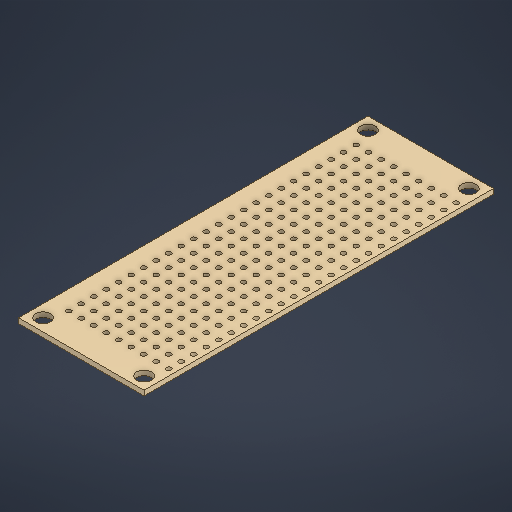
# Autodesk Inventor part: perfboard-71x51x1
Saved by Autodesk Inventor 2025.2 (Build 292293000, 293)
## iProperties
Created: 2025-11-15
Part Number: perfboard-71x51x1
Material: Fiberglass Batt
Document SubType Name: Modeling
Designer: sam
Density: 0.032 g/cm^3
Appearance: Golden Sand
Author: sam
Autodesk Inventor part; units mm, degrees
ref_plane "YZ Plane" through (0, 0, 0) normal (1, 0, 0) x (0, 1, 0)
ref_plane "XZ Plane" through (0, 0, 0) normal (0, 1, 0) x (-1, 0, 0)
ref_plane "XY Plane" through (0, 0, 0) normal (0, 0, 1) x (1, 0, 0)
sketch "Sketch1" plane through (0, 0, 0) normal (0, 1, 0) x (-1, 0, 0)
  line L0 (-12.75, -35.5) -> (12.75, -35.5)
  line L1 (12.75, -35.5) -> (12.75, 35.5)
  line L2 (12.75, 35.5) -> (-12.75, 35.5)
  line L3 (-12.75, 35.5) -> (-12.75, -35.5)
  line L4 (-12.75, -35.5) -> (12.75, 35.5) construction
  line L5 (12.75, -35.5) -> (-12.75, 35.5) construction
  circle A0 centre (8.84, -29.21) radius 0.5
  circle A1 centre (6.3, -29.21) radius 0.5
  circle A2 centre (3.76, -29.21) radius 0.5
  circle A3 centre (1.22, -29.21) radius 0.5
  circle A4 centre (-1.32, -29.21) radius 0.5
  circle A5 centre (-3.86, -29.21) radius 0.5
  circle A6 centre (-6.4, -29.21) radius 0.5
  circle A7 centre (-8.94, -29.21) radius 0.5
  circle A8 centre (-11.48, -29.21) radius 0.5
  circle A9 centre (8.84, -26.67) radius 0.5
  circle A10 centre (6.3, -26.67) radius 0.5
  circle A11 centre (3.76, -26.67) radius 0.5
  circle A12 centre (1.22, -26.67) radius 0.5
  circle A13 centre (-1.32, -26.67) radius 0.5
  circle A14 centre (-3.86, -26.67) radius 0.5
  circle A15 centre (-6.4, -26.67) radius 0.5
  circle A16 centre (-8.94, -26.67) radius 0.5
  circle A17 centre (-11.48, -26.67) radius 0.5
  circle A18 centre (8.84, -24.13) radius 0.5
  circle A19 centre (6.3, -24.13) radius 0.5
  circle A20 centre (3.76, -24.13) radius 0.5
  circle A21 centre (1.22, -24.13) radius 0.5
  circle A22 centre (-1.32, -24.13) radius 0.5
  circle A23 centre (-3.86, -24.13) radius 0.5
  circle A24 centre (-6.4, -24.13) radius 0.5
  circle A25 centre (-8.94, -24.13) radius 0.5
  circle A26 centre (-11.48, -24.13) radius 0.5
  circle A27 centre (8.84, -21.59) radius 0.5
  circle A28 centre (6.3, -21.59) radius 0.5
  circle A29 centre (3.76, -21.59) radius 0.5
  circle A30 centre (1.22, -21.59) radius 0.5
  circle A31 centre (-1.32, -21.59) radius 0.5
  circle A32 centre (-3.86, -21.59) radius 0.5
  circle A33 centre (-6.4, -21.59) radius 0.5
  circle A34 centre (-8.94, -21.59) radius 0.5
  circle A35 centre (-11.48, -21.59) radius 0.5
  circle A36 centre (8.84, -19.05) radius 0.5
  circle A37 centre (6.3, -19.05) radius 0.5
  circle A38 centre (3.76, -19.05) radius 0.5
  circle A39 centre (1.22, -19.05) radius 0.5
  circle A40 centre (-1.32, -19.05) radius 0.5
  circle A41 centre (-3.86, -19.05) radius 0.5
  circle A42 centre (-6.4, -19.05) radius 0.5
  circle A43 centre (-8.94, -19.05) radius 0.5
  circle A44 centre (-11.48, -19.05) radius 0.5
  circle A45 centre (8.84, -16.51) radius 0.5
  circle A46 centre (6.3, -16.51) radius 0.5
  circle A47 centre (3.76, -16.51) radius 0.5
  circle A48 centre (1.22, -16.51) radius 0.5
  circle A49 centre (-1.32, -16.51) radius 0.5
  circle A50 centre (-3.86, -16.51) radius 0.5
  circle A51 centre (-6.4, -16.51) radius 0.5
  circle A52 centre (-8.94, -16.51) radius 0.5
  circle A53 centre (-11.48, -16.51) radius 0.5
  circle A54 centre (8.84, -13.97) radius 0.5
  circle A55 centre (6.3, -13.97) radius 0.5
  circle A56 centre (3.76, -13.97) radius 0.5
  circle A57 centre (1.22, -13.97) radius 0.5
  circle A58 centre (-1.32, -13.97) radius 0.5
  circle A59 centre (-3.86, -13.97) radius 0.5
  circle A60 centre (-6.4, -13.97) radius 0.5
  circle A61 centre (-8.94, -13.97) radius 0.5
  circle A62 centre (-11.48, -13.97) radius 0.5
  circle A63 centre (8.84, -11.43) radius 0.5
  circle A64 centre (6.3, -11.43) radius 0.5
  circle A65 centre (3.76, -11.43) radius 0.5
  circle A66 centre (1.22, -11.43) radius 0.5
  circle A67 centre (-1.32, -11.43) radius 0.5
  circle A68 centre (-3.86, -11.43) radius 0.5
  circle A69 centre (-6.4, -11.43) radius 0.5
  circle A70 centre (-8.94, -11.43) radius 0.5
  circle A71 centre (-11.48, -11.43) radius 0.5
  circle A72 centre (8.84, -8.89) radius 0.5
  circle A73 centre (6.3, -8.89) radius 0.5
  circle A74 centre (3.76, -8.89) radius 0.5
  circle A75 centre (1.22, -8.89) radius 0.5
  circle A76 centre (-1.32, -8.89) radius 0.5
  circle A77 centre (-3.86, -8.89) radius 0.5
  circle A78 centre (-6.4, -8.89) radius 0.5
  circle A79 centre (-8.94, -8.89) radius 0.5
  circle A80 centre (-11.48, -8.89) radius 0.5
  circle A81 centre (8.84, -6.35) radius 0.5
  circle A82 centre (6.3, -6.35) radius 0.5
  circle A83 centre (3.76, -6.35) radius 0.5
  circle A84 centre (1.22, -6.35) radius 0.5
  circle A85 centre (-1.32, -6.35) radius 0.5
  circle A86 centre (-3.86, -6.35) radius 0.5
  circle A87 centre (-6.4, -6.35) radius 0.5
  circle A88 centre (-8.94, -6.35) radius 0.5
  circle A89 centre (-11.48, -6.35) radius 0.5
  circle A90 centre (8.84, -3.81) radius 0.5
  circle A91 centre (6.3, -3.81) radius 0.5
  circle A92 centre (3.76, -3.81) radius 0.5
  circle A93 centre (1.22, -3.81) radius 0.5
  circle A94 centre (-1.32, -3.81) radius 0.5
  circle A95 centre (-3.86, -3.81) radius 0.5
  circle A96 centre (-6.4, -3.81) radius 0.5
  circle A97 centre (-8.94, -3.81) radius 0.5
  circle A98 centre (-11.48, -3.81) radius 0.5
  circle A99 centre (8.84, -1.27) radius 0.5
  circle A100 centre (6.3, -1.27) radius 0.5
  circle A101 centre (3.76, -1.27) radius 0.5
  circle A102 centre (1.22, -1.27) radius 0.5
  circle A103 centre (-1.32, -1.27) radius 0.5
  circle A104 centre (-3.86, -1.27) radius 0.5
  circle A105 centre (-6.4, -1.27) radius 0.5
  circle A106 centre (-8.94, -1.27) radius 0.5
  circle A107 centre (-11.48, -1.27) radius 0.5
  circle A108 centre (8.84, 1.27) radius 0.5
  circle A109 centre (6.3, 1.27) radius 0.5
  circle A110 centre (3.76, 1.27) radius 0.5
  circle A111 centre (1.22, 1.27) radius 0.5
  circle A112 centre (-1.32, 1.27) radius 0.5
  circle A113 centre (-3.86, 1.27) radius 0.5
  circle A114 centre (-6.4, 1.27) radius 0.5
  circle A115 centre (-8.94, 1.27) radius 0.5
  circle A116 centre (-11.48, 1.27) radius 0.5
  circle A117 centre (8.84, 3.81) radius 0.5
  circle A118 centre (6.3, 3.81) radius 0.5
  circle A119 centre (3.76, 3.81) radius 0.5
  circle A120 centre (1.22, 3.81) radius 0.5
  circle A121 centre (-1.32, 3.81) radius 0.5
  circle A122 centre (-3.86, 3.81) radius 0.5
  circle A123 centre (-6.4, 3.81) radius 0.5
  circle A124 centre (-8.94, 3.81) radius 0.5
  circle A125 centre (-11.48, 3.81) radius 0.5
  circle A126 centre (8.84, 6.35) radius 0.5
  circle A127 centre (6.3, 6.35) radius 0.5
  circle A128 centre (3.76, 6.35) radius 0.5
  circle A129 centre (1.22, 6.35) radius 0.5
  circle A130 centre (-1.32, 6.35) radius 0.5
  circle A131 centre (-3.86, 6.35) radius 0.5
  circle A132 centre (-6.4, 6.35) radius 0.5
  circle A133 centre (-8.94, 6.35) radius 0.5
  circle A134 centre (-11.48, 6.35) radius 0.5
  circle A135 centre (8.84, 8.89) radius 0.5
  circle A136 centre (6.3, 8.89) radius 0.5
  circle A137 centre (3.76, 8.89) radius 0.5
  circle A138 centre (1.22, 8.89) radius 0.5
  circle A139 centre (-1.32, 8.89) radius 0.5
  circle A140 centre (-3.86, 8.89) radius 0.5
  circle A141 centre (-6.4, 8.89) radius 0.5
  circle A142 centre (-8.94, 8.89) radius 0.5
  circle A143 centre (-11.48, 8.89) radius 0.5
  circle A144 centre (8.84, 11.43) radius 0.5
  circle A145 centre (6.3, 11.43) radius 0.5
  circle A146 centre (3.76, 11.43) radius 0.5
  circle A147 centre (1.22, 11.43) radius 0.5
  circle A148 centre (-1.32, 11.43) radius 0.5
  circle A149 centre (-3.86, 11.43) radius 0.5
  circle A150 centre (-6.4, 11.43) radius 0.5
  circle A151 centre (-8.94, 11.43) radius 0.5
  circle A152 centre (-11.48, 11.43) radius 0.5
  circle A153 centre (8.84, 13.97) radius 0.5
  circle A154 centre (6.3, 13.97) radius 0.5
  circle A155 centre (3.76, 13.97) radius 0.5
  circle A156 centre (1.22, 13.97) radius 0.5
  circle A157 centre (-1.32, 13.97) radius 0.5
  circle A158 centre (-3.86, 13.97) radius 0.5
  circle A159 centre (-6.4, 13.97) radius 0.5
  circle A160 centre (-8.94, 13.97) radius 0.5
  circle A161 centre (-11.48, 13.97) radius 0.5
  circle A162 centre (8.84, 16.51) radius 0.5
  circle A163 centre (6.3, 16.51) radius 0.5
  circle A164 centre (3.76, 16.51) radius 0.5
  circle A165 centre (1.22, 16.51) radius 0.5
  circle A166 centre (-1.32, 16.51) radius 0.5
  circle A167 centre (-3.86, 16.51) radius 0.5
  circle A168 centre (-6.4, 16.51) radius 0.5
  circle A169 centre (-8.94, 16.51) radius 0.5
  circle A170 centre (-11.48, 16.51) radius 0.5
  circle A171 centre (8.84, 19.05) radius 0.5
  circle A172 centre (6.3, 19.05) radius 0.5
  circle A173 centre (3.76, 19.05) radius 0.5
  circle A174 centre (1.22, 19.05) radius 0.5
  circle A175 centre (-1.32, 19.05) radius 0.5
  circle A176 centre (-3.86, 19.05) radius 0.5
  circle A177 centre (-6.4, 19.05) radius 0.5
  circle A178 centre (-8.94, 19.05) radius 0.5
  circle A179 centre (-11.48, 19.05) radius 0.5
  circle A180 centre (8.84, 21.59) radius 0.5
  circle A181 centre (6.3, 21.59) radius 0.5
  circle A182 centre (3.76, 21.59) radius 0.5
  circle A183 centre (1.22, 21.59) radius 0.5
  circle A184 centre (-1.32, 21.59) radius 0.5
  circle A185 centre (-3.86, 21.59) radius 0.5
  circle A186 centre (-6.4, 21.59) radius 0.5
  circle A187 centre (-8.94, 21.59) radius 0.5
  circle A188 centre (-11.48, 21.59) radius 0.5
  circle A189 centre (8.84, 24.13) radius 0.5
  circle A190 centre (6.3, 24.13) radius 0.5
  circle A191 centre (3.76, 24.13) radius 0.5
  circle A192 centre (1.22, 24.13) radius 0.5
  circle A193 centre (-1.32, 24.13) radius 0.5
  circle A194 centre (-3.86, 24.13) radius 0.5
  circle A195 centre (-6.4, 24.13) radius 0.5
  circle A196 centre (-8.94, 24.13) radius 0.5
  circle A197 centre (-11.48, 24.13) radius 0.5
  circle A198 centre (8.84, 26.67) radius 0.5
  circle A199 centre (6.3, 26.67) radius 0.5
  circle A200 centre (3.76, 26.67) radius 0.5
  circle A201 centre (1.22, 26.67) radius 0.5
  circle A202 centre (-1.32, 26.67) radius 0.5
  circle A203 centre (-3.86, 26.67) radius 0.5
  circle A204 centre (-6.4, 26.67) radius 0.5
  circle A205 centre (-8.94, 26.67) radius 0.5
  circle A206 centre (-11.48, 26.67) radius 0.5
  circle A207 centre (8.84, 29.21) radius 0.5
  circle A208 centre (6.3, 29.21) radius 0.5
  circle A209 centre (3.76, 29.21) radius 0.5
  circle A210 centre (1.22, 29.21) radius 0.5
  circle A211 centre (-1.32, 29.21) radius 0.5
  circle A212 centre (-3.86, 29.21) radius 0.5
  circle A213 centre (-6.4, 29.21) radius 0.5
  circle A214 centre (-8.94, 29.21) radius 0.5
  circle A215 centre (-11.48, 29.21) radius 0.5
  circle A216 centre (-10.25, -33) radius 1.5
  circle A217 centre (-10.25, 33) radius 1.5
  circle A218 centre (10.25, 33) radius 1.5
  circle A219 centre (10.25, -33) radius 1.5
  point P0 (0, 0)
  dimension "d0" = 25.5
  dimension "d1" = 71
  dimension "d2" = 1
  dimension "d5" = 2.54
  dimension "d8" = 2.54
  dimension "d11" = 6.29
  dimension "d12" = 3.91
  dimension "d13" = 3
  dimension "d14" = 2.5
  dimension "d15" = 2.5
  dimension "d16" = 3
  dimension "d17" = 2.5
  dimension "d18" = 2.5
  dimension "d19" = 3
  dimension "d20" = 2.5
  dimension "d21" = 2.5
  dimension "d22" = 3
  dimension "d23" = 2.5
  dimension "d24" = 2.5
  constraints: 220 centre point, 12 end point, 2 horizontal, 2 midpoint, 2 parallel, 1 perpendicular, 1 vertical, 430 other
  measures "d0" distance of L2.end L1.end
  measures "d1" distance of L1.end L0.end
  measures "d2" diameter of A0
  measures "d5" distance of A0.centre A1.centre
  measures "d8" distance of A0.centre A9.centre
  measures "d11" distance from line of L0 A0.centre
  measures "d12" distance from line of L1 A0.centre
  measures "d13" diameter of A216
  measures "d14" distance from line of L0 A216.centre
  measures "d15" distance from line of L3 A216.centre
  measures "d16" diameter of A217
  measures "d17" distance from line of L3 A217.centre
  measures "d18" distance from line of L2 A217.centre
  measures "d19" diameter of A218
  measures "d20" distance from line of L2 A218.centre
  measures "d21" distance from line of L1 A218.centre
  measures "d22" diameter of A219
  measures "d23" distance from line of L1 A219.centre
  measures "d24" distance from line of L0 A219.centre
extrude "Extrusion1" add sketch "Sketch1" along normal blind 1
body "Solid1"
